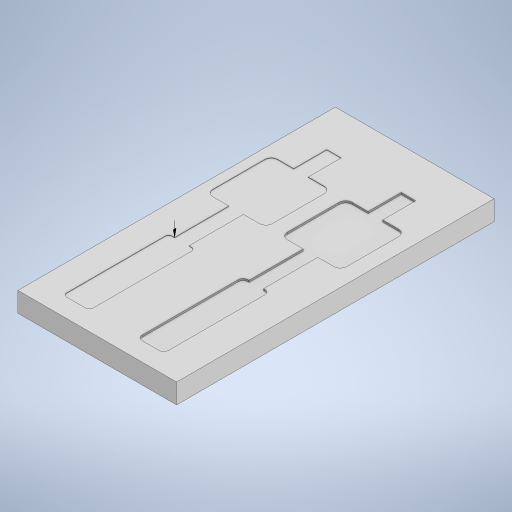
# Autodesk Inventor part: 0p03_total_thickness
Saved by Autodesk Inventor 2024.2 (Build 282272000, 272)
## iProperties
Created: 2024-10-29
Part Number: 0p03_total_thickness
Material: Generic
Document SubType Name: Modeling
Designer: Tom
Density: 1 g/cm^3
Appearance: Default
Author: Tom
Autodesk Inventor part; units mm, degrees
ref_plane "YZ Plane" through (0, 0, 0) normal (1, 0, 0) x (0, 1, 0)
ref_plane "XZ Plane" through (0, 0, 0) normal (0, 1, 0) x (-1, 0, 0)
ref_plane "XY Plane" through (0, 0, 0) normal (0, 0, 1) x (1, 0, 0)
sketch "Sketch1" plane through (0, 0, 0) normal (0, 1, 0) x (-1, 0, 0)
  line L0 (0, 0) -> (76.2, 0)
  line L1 (76.2, 0) -> (76.2, -152.4)
  line L2 (76.2, -152.4) -> (0, -152.4)
  line L3 (0, -152.4) -> (0, 0)
  dimension "d0" = 76.2
  dimension "d1" = 152.4
  constraints: 8 end point, 2 parallel, 1 horizontal, 1 perpendicular
  measures "d0" distance of L0.start L0.end
  measures "d1" distance of L2.end L0.start
extrude "Extrusion1" add sketch "Sketch1" along normal blind 9.525
sketch "Sketch2" plane through (0, 9.525, 0) normal (0, 1, 0) x (1, 0, 0)
  line L0 (-61.7538, 8.89) -> (-52.5462, 8.89)
  line L1 (-50.8, 10.6362) -> (-50.8, 57.9438)
  line L2 (-63.5, 57.9438) -> (-63.5, 10.6362)
  line L3 (-76.2, 152.4) -> (-76.2, 0) projected
  line L4 (-76.2, 0) -> (0, 0) projected
  arc A0 (-63.5, 10.6362) -> (-61.7538, 8.89) centre (-61.7538, 10.6362) ccw
  arc A1 (-52.5462, 8.89) -> (-50.8, 10.6362) centre (-52.5462, 10.6362) ccw
  arc A2 (-50.8, 57.9438) -> (-52.5462, 59.69) centre (-52.5462, 57.9438) ccw
  arc A3 (-61.7538, 59.69) -> (-63.5, 57.9438) centre (-61.7538, 57.9438) ccw
  line L5 (-60.6425, 59.69) -> (-53.6575, 59.69)
  line L6 (-53.6575, 59.69) -> (-53.6575, 132.715)
  line L7 (-53.6575, 132.715) -> (-60.6425, 132.715)
  line L8 (-60.6425, 132.715) -> (-60.6425, 59.69)
  line L9 (-52.5462, 59.69) -> (-53.6575, 59.69)
  line L10 (-60.6425, 59.69) -> (-61.7538, 59.69)
  line L11 (-68.2625, 116.84) -> (-46.0375, 116.84)
  line L12 (-42.8625, 113.665) -> (-42.8625, 88.9)
  line L13 (-46.0375, 85.725) -> (-68.2625, 85.725)
  line L14 (-71.4375, 88.9) -> (-71.4375, 113.665)
  arc A4 (-71.4375, 88.9) -> (-68.2625, 85.725) centre (-68.2625, 88.9) ccw
  arc A5 (-68.2625, 116.84) -> (-71.4375, 113.665) centre (-68.2625, 113.665) ccw
  arc A6 (-42.8625, 113.665) -> (-46.0375, 116.84) centre (-46.0375, 113.665) ccw
  arc A7 (-46.0375, 85.725) -> (-42.8625, 88.9) centre (-46.0375, 88.9) ccw
  point P0 (-63.5, 8.89)
  point P1 (-50.8, 69.85)
  point P2 (-50.8, 8.89)
  point P3 (-63.5, 69.85)
  point P4 (-57.15, 69.85)
  point P5 (-57.15, 132.715)
  point P6 (-71.4375, 116.84)
  point P7 (-42.8625, 85.725)
  point P8 (-42.8625, 116.84)
  point P9 (-71.4375, 85.725)
  point P10 (-57.15, 116.84)
  point P11 (-57.15, 8.89)
  point P12 (-57.15, 59.69)
  point P13 (-60.6425, 85.725)
  point P14 (-60.6425, 116.84)
  point P15 (-53.6575, 116.84)
  point P16 (-53.6575, 85.725)
  dimension "d22" = 0
  dimension "d28" = 0
  dimension "d36" = 26.035
  dimension "d37" = 50.8
  constraints: 26 end point, 18 tangent, 16 point on circle, 14 point on line, 8 centre point, 7 parallel, 6 equal radius, 4 midpoint, 3 horizontal, 3 perpendicular
  measures "d22" horizontal distance of point (-57.15, 69.85) point (-57.15, 132.715)
  measures "d28" horizontal distance of point (-57.15, 8.89) point (-57.15, 59.69)
  measures "d36" distance between parallel lines of L5 L13
  measures "d37" distance between parallel lines of L0 L5
extrude "Extrusion2" cut sketch "Sketch2" against normal blind 0.254
sketch "Sketch3" plane through (0, 9.525, 0) normal (0, 1, 0) x (1, 0, 0)
  line L0 (-25.3994, 8.89) -> (-17.4619, 8.89)
  line L1 (-15.0807, 11.2712) -> (-15.0807, 57.3087)
  line L2 (-27.7807, 57.3087) -> (-27.7807, 11.2712)
  arc A0 (-27.7807, 11.2712) -> (-25.3994, 8.89) centre (-25.3994, 11.2712) ccw
  arc A1 (-17.4619, 8.89) -> (-15.0807, 11.2712) centre (-17.4619, 11.2712) ccw
  arc A2 (-15.0807, 57.3087) -> (-17.4619, 59.69) centre (-17.4619, 57.3087) ccw
  arc A3 (-25.3994, 59.69) -> (-27.7807, 57.3087) centre (-25.3994, 57.3087) ccw
  line L3 (-17.9382, 59.69) -> (-17.9382, 132.715)
  line L4 (-17.9382, 132.715) -> (-24.9232, 132.715)
  line L5 (-24.9232, 132.715) -> (-24.9232, 59.69)
  line L6 (0, 152.4) -> (-76.2, 152.4) projected
  line L7 (-17.4619, 59.69) -> (-17.9382, 59.69)
  line L8 (-24.9232, 59.69) -> (-25.3994, 59.69)
  line L9 (-32.5432, 116.84) -> (-10.3182, 116.84)
  line L10 (-7.1432, 113.665) -> (-7.1432, 88.9)
  line L11 (-10.3182, 85.725) -> (-32.5432, 85.725)
  line L12 (-35.7182, 88.9) -> (-35.7182, 113.665)
  line L13 (-46.0375, 85.725) -> (-53.6575, 85.725) projected
  arc A4 (-32.5432, 116.84) -> (-35.7182, 113.665) centre (-32.5432, 113.665) ccw
  arc A5 (-35.7182, 88.9) -> (-32.5432, 85.725) centre (-32.5432, 88.9) ccw
  arc A6 (-10.3182, 85.725) -> (-7.1432, 88.9) centre (-10.3182, 88.9) ccw
  arc A7 (-7.1432, 113.665) -> (-10.3182, 116.84) centre (-10.3182, 113.665) ccw
  point P0 (0, 0)
  point P1 (-27.7807, 8.89)
  point P2 (-27.7807, 59.69)
  point P3 (-21.4307, 55.0791)
  point P4 (-21.4307, 132.715)
  point P5 (-7.1432, 85.725)
  point P6 (-35.7182, 85.725)
  point P7 (-21.4307, 116.84)
  point P8 (-49.8475, 85.725)
  point P9 (-24.9232, 85.725)
  point P10 (-24.9232, 116.84)
  point P11 (-17.9382, 116.84)
  point P12 (-17.9382, 85.725)
  point P13 (-25.1613, 59.69)
  dimension "d11" = 50.8
  dimension "d12" = 12.7
  dimension "d13" = 2.3813
  dimension "d17" = 0
  dimension "d20" = 73.025
  dimension "d33" = 0
  dimension "d34" = 3.175
  dimension "d40" = 26.035
  constraints: 24 end point, 18 tangent, 16 point on circle, 8 centre point, 7 point on line, 6 equal radius, 6 parallel, 4 midpoint, 2 horizontal, 2 perpendicular
  measures "d11" distance of point (-27.781, 59.69) point (-27.781, 8.89)
  measures "d12" distance between parallel lines of L1 L2
  measures "d13" radius of A0
  measures "d17" horizontal distance of point (-21.431, 55.079) point (-21.431, 132.715)
  measures "d20" distance of L4.end L5.end
  measures "d33" distance from line of point (-49.847, 85.725) L11
  measures "d34" radius of A4
  measures "d40" distance from line of L11 point (-25.161, 59.69)
extrude "Extrusion3" cut sketch "Sketch3" against normal blind 0.889
body "Solid1"
